Autodesk Fusion 360 part; units mm, degrees
(part 7 of 10)
sketch "草图24 (3)" plane through (0, 0, 0) normal (0, 0, 1) x (1, 0, 0) in component "R2_Integrated"
  line L0 (729, 50) -> (737, 50)
  line L1 (737, 50) -> (737, 131)
  line L2 (737, 131) -> (729, 131)
  line L3 (729, 131) -> (729, 50)
  dimension "d2854" = 729
  dimension "d2855" = 50
  dimension "d2856" = 8
  dimension "d2857" = 81
  constraint horizontal L0
  constraint vertical L1
  constraint horizontal L2
  constraint vertical L3
  measures "d2854" horizontal distance of origin L0.start
  measures "d2855" vertical distance of origin L0.start
  measures "d2856" horizontal distance of L0.start L0.end
  measures "d2857" vertical distance of L0.end L1.end
extrude "R03 integral runner 0''" add sketch "草图24 (3)" along normal blind 20 bodies 19 in component "R2_Integrated"
ref_plane "工作平面25" through (0, 0, 0) normal (0, 0, 1) x (1, 0, 0) in component "R2_Integrated"
sketch "草图25 (3)" plane through (0, 0, 0) normal (0, 0, 1) x (1, 0, 0) in component "R2_Integrated"
  line L0 (849, 50) -> (857, 50)
  line L1 (857, 50) -> (857, 131)
  line L2 (857, 131) -> (849, 131)
  line L3 (849, 131) -> (849, 50)
  dimension "d2862" = 849
  dimension "d2863" = 50
  dimension "d2864" = 8
  dimension "d2865" = 81
  constraint horizontal L0
  constraint vertical L1
  constraint horizontal L2
  constraint vertical L3
  measures "d2862" horizontal distance of origin L0.start
  measures "d2863" vertical distance of origin L0.start
  measures "d2864" horizontal distance of L0.start L0.end
  measures "d2865" vertical distance of L0.end L1.end
extrude "R03 integral runner 1''" add sketch "草图25 (3)" along normal blind 20 bodies 19 in component "R2_Integrated"
chamfer "R03 touch edge chamfer'''" distance 0.4 angle 45 5 edges at (729, 102.5, 40) (793, 53, 40) (857, 102.5, 40) (726, 95, 40) (860, 95, 40) on bodies 19 in component "R2_Integrated"
ref_plane "工作平面20" through (0, 0, 20) normal (0, 0, 1) x (1, 0, 0) in component "LS_Integrated"
sketch "草图20 (7)" plane through (0, 0, 20) normal (0, 0, 1) x (1, 0, 0) in component "LS_Integrated"
  line L0 (56.75, 306.75) -> (65.25, 306.75)
  line L1 (65.25, 306.75) -> (65.25, 315.25)
  line L2 (65.25, 315.25) -> (56.75, 315.25)
  line L3 (56.75, 315.25) -> (56.75, 306.75)
  dimension "d2871" = 56.75
  dimension "d2872" = 306.75
  dimension "d2873" = 8.5
  dimension "d2874" = 8.5
  constraint horizontal L0
  constraint vertical L1
  constraint horizontal L2
  constraint vertical L3
  measures "d2871" horizontal distance of origin L0.start
  measures "d2872" vertical distance of origin L0.start
  measures "d2873" horizontal distance of L0.start L0.end
  measures "d2874" vertical distance of L0.end L1.end
extrude "R03 fill obsolete socket 00''''" add sketch "草图20 (7)" along normal blind 1.8 bodies 25 in component "LS_Integrated"
ref_plane "工作平面21" through (0, 0, 20) normal (0, 0, 1) x (1, 0, 0) in component "LS_Integrated"
sketch "草图21 (7)" plane through (0, 0, 20) normal (0, 0, 1) x (1, 0, 0) in component "LS_Integrated"
  line L0 (148.75, 306.75) -> (157.25, 306.75)
  line L1 (157.25, 306.75) -> (157.25, 315.25)
  line L2 (157.25, 315.25) -> (148.75, 315.25)
  line L3 (148.75, 315.25) -> (148.75, 306.75)
  dimension "d2879" = 148.75
  dimension "d2880" = 306.75
  dimension "d2881" = 8.5
  dimension "d2882" = 8.5
  constraint horizontal L0
  constraint vertical L1
  constraint horizontal L2
  constraint vertical L3
  measures "d2879" horizontal distance of origin L0.start
  measures "d2880" vertical distance of origin L0.start
  measures "d2881" horizontal distance of L0.start L0.end
  measures "d2882" vertical distance of L0.end L1.end
extrude "R03 fill obsolete socket 01''''" add sketch "草图21 (7)" along normal blind 1.8 bodies 25 in component "LS_Integrated"
ref_plane "工作平面22" through (0, 0, 20) normal (0, 0, 1) x (1, 0, 0) in component "LS_Integrated"
sketch "草图22 (6)" plane through (0, 0, 20) normal (0, 0, 1) x (1, 0, 0) in component "LS_Integrated"
  line L0 (56.75, 148.75) -> (65.25, 148.75)
  line L1 (65.25, 148.75) -> (65.25, 157.25)
  line L2 (65.25, 157.25) -> (56.75, 157.25)
  line L3 (56.75, 157.25) -> (56.75, 148.75)
  dimension "d2887" = 56.75
  dimension "d2888" = 148.75
  dimension "d2889" = 8.5
  dimension "d2890" = 8.5
  constraint horizontal L0
  constraint vertical L1
  constraint horizontal L2
  constraint vertical L3
  measures "d2887" horizontal distance of origin L0.start
  measures "d2888" vertical distance of origin L0.start
  measures "d2889" horizontal distance of L0.start L0.end
  measures "d2890" vertical distance of L0.end L1.end
extrude "R03 fill obsolete socket 10''''" add sketch "草图22 (6)" along normal blind 1.8 bodies 25 in component "LS_Integrated"
ref_plane "工作平面23" through (0, 0, 20) normal (0, 0, 1) x (1, 0, 0) in component "LS_Integrated"
sketch "草图23 (6)" plane through (0, 0, 20) normal (0, 0, 1) x (1, 0, 0) in component "LS_Integrated"
  line L0 (148.75, 148.75) -> (157.25, 148.75)
  line L1 (157.25, 148.75) -> (157.25, 157.25)
  line L2 (157.25, 157.25) -> (148.75, 157.25)
  line L3 (148.75, 157.25) -> (148.75, 148.75)
  dimension "d2895" = 148.75
  dimension "d2896" = 148.75
  dimension "d2897" = 8.5
  dimension "d2898" = 8.5
  constraint horizontal L0
  constraint vertical L1
  constraint horizontal L2
  constraint vertical L3
  measures "d2895" horizontal distance of origin L0.start
  measures "d2896" vertical distance of origin L0.start
  measures "d2897" horizontal distance of L0.start L0.end
  measures "d2898" vertical distance of L0.end L1.end
extrude "R03 fill obsolete socket 11''''" add sketch "草图23 (6)" along normal blind 1.8 bodies 25 in component "LS_Integrated"
ref_plane "工作平面24" through (0, 0, 0) normal (0, 0, 1) x (1, 0, 0) in component "LS_Integrated"
sketch "草图24 (4)" plane through (0, 0, 0) normal (0, 0, 1) x (1, 0, 0) in component "LS_Integrated"
  line L0 (50, 311) -> (161, 311)
  line L1 (161, 311) -> (161, 319)
  line L2 (161, 319) -> (50, 319)
  line L3 (50, 319) -> (50, 311)
  dimension "d2903" = 50
  dimension "d2904" = 311
  dimension "d2905" = 111
  dimension "d2906" = 8
  constraint horizontal L0
  constraint vertical L1
  constraint horizontal L2
  constraint vertical L3
  measures "d2903" horizontal distance of origin L0.start
  measures "d2904" vertical distance of origin L0.start
  measures "d2905" horizontal distance of L0.start L0.end
  measures "d2906" vertical distance of L0.end L1.end
extrude "R03 integral runner 0'''" add sketch "草图24 (4)" along normal blind 20 bodies 25 in component "LS_Integrated"
ref_plane "工作平面25" through (0, 0, 0) normal (0, 0, 1) x (1, 0, 0) in component "LS_Integrated"
sketch "草图25 (4)" plane through (0, 0, 0) normal (0, 0, 1) x (1, 0, 0) in component "LS_Integrated"
  line L0 (50, 145) -> (161, 145)
  line L1 (161, 145) -> (161, 153)
  line L2 (161, 153) -> (50, 153)
  line L3 (50, 153) -> (50, 145)
  dimension "d2911" = 50
  dimension "d2912" = 145
  dimension "d2913" = 111
  dimension "d2914" = 8
  constraint horizontal L0
  constraint vertical L1
  constraint horizontal L2
  constraint vertical L3
  measures "d2911" horizontal distance of origin L0.start
  measures "d2912" vertical distance of origin L0.start
  measures "d2913" horizontal distance of L0.start L0.end
  measures "d2914" vertical distance of L0.end L1.end
extrude "R03 integral runner 1'''" add sketch "草图25 (4)" along normal blind 20 bodies 25 in component "LS_Integrated"
chamfer "R03 touch edge chamfer''''" distance 0.4 angle 45 5 edges at (117.5, 145, 40) (117.5, 319, 40) (110, 322, 40) (110, 142, 40) (53, 232, 40) on bodies 25 in component "LS_Integrated"
ref_plane "工作平面20" through (0, 0, 20) normal (0, 0, 1) x (1, 0, 0) in component "RS_Integrated"
sketch "草图20 (8)" plane through (0, 0, 20) normal (0, 0, 1) x (1, 0, 0) in component "RS_Integrated"
  line L0 (844.75, 148.75) -> (853.25, 148.75)
  line L1 (853.25, 148.75) -> (853.25, 157.25)
  line L2 (853.25, 157.25) -> (844.75, 157.25)
  line L3 (844.75, 157.25) -> (844.75, 148.75)
  dimension "d2920" = 844.75
  dimension "d2921" = 148.75
  dimension "d2922" = 8.5
  dimension "d2923" = 8.5
  constraint horizontal L0
  constraint vertical L1
  constraint horizontal L2
  constraint vertical L3
  measures "d2920" horizontal distance of origin L0.start
  measures "d2921" vertical distance of origin L0.start
  measures "d2922" horizontal distance of L0.start L0.end
  measures "d2923" vertical distance of L0.end L1.end
extrude "R03 fill obsolete socket 00'''''" add sketch "草图20 (8)" along normal blind 1.8 bodies 31 in component "RS_Integrated"
ref_plane "工作平面21" through (0, 0, 20) normal (0, 0, 1) x (1, 0, 0) in component "RS_Integrated"
sketch "草图21 (8)" plane through (0, 0, 20) normal (0, 0, 1) x (1, 0, 0) in component "RS_Integrated"
  line L0 (782.75, 148.75) -> (791.25, 148.75)
  line L1 (791.25, 148.75) -> (791.25, 157.25)
  line L2 (791.25, 157.25) -> (782.75, 157.25)
  line L3 (782.75, 157.25) -> (782.75, 148.75)
  dimension "d2928" = 782.75
  dimension "d2929" = 148.75
  dimension "d2930" = 8.5
  dimension "d2931" = 8.5
  constraint horizontal L0
  constraint vertical L1
  constraint horizontal L2
  constraint vertical L3
  measures "d2928" horizontal distance of origin L0.start
  measures "d2929" vertical distance of origin L0.start
  measures "d2930" horizontal distance of L0.start L0.end
  measures "d2931" vertical distance of L0.end L1.end
extrude "R03 fill obsolete socket 01'''''" add sketch "草图21 (8)" along normal blind 1.8 bodies 31 in component "RS_Integrated"
ref_plane "工作平面22" through (0, 0, 20) normal (0, 0, 1) x (1, 0, 0) in component "RS_Integrated"
sketch "草图22 (7)" plane through (0, 0, 20) normal (0, 0, 1) x (1, 0, 0) in component "RS_Integrated"
  line L0 (844.75, 306.75) -> (853.25, 306.75)
  line L1 (853.25, 306.75) -> (853.25, 315.25)
  line L2 (853.25, 315.25) -> (844.75, 315.25)
  line L3 (844.75, 315.25) -> (844.75, 306.75)
  dimension "d2936" = 844.75
  dimension "d2937" = 306.75
  dimension "d2938" = 8.5
  dimension "d2939" = 8.5
  constraint horizontal L0
  constraint vertical L1
  constraint horizontal L2
  constraint vertical L3
  measures "d2936" horizontal distance of origin L0.start
  measures "d2937" vertical distance of origin L0.start
  measures "d2938" horizontal distance of L0.start L0.end
  measures "d2939" vertical distance of L0.end L1.end
extrude "R03 fill obsolete socket 10'''''" add sketch "草图22 (7)" along normal blind 1.8 bodies 31 in component "RS_Integrated"
ref_plane "工作平面23" through (0, 0, 20) normal (0, 0, 1) x (1, 0, 0) in component "RS_Integrated"
sketch "草图23 (7)" plane through (0, 0, 20) normal (0, 0, 1) x (1, 0, 0) in component "RS_Integrated"
  line L0 (782.75, 306.75) -> (791.25, 306.75)
  line L1 (791.25, 306.75) -> (791.25, 315.25)
  line L2 (791.25, 315.25) -> (782.75, 315.25)
  line L3 (782.75, 315.25) -> (782.75, 306.75)
  dimension "d2944" = 782.75
  dimension "d2945" = 306.75
  dimension "d2946" = 8.5
  dimension "d2947" = 8.5
  constraint horizontal L0
  constraint vertical L1
  constraint horizontal L2
  constraint vertical L3
  measures "d2944" horizontal distance of origin L0.start
  measures "d2945" vertical distance of origin L0.start
  measures "d2946" horizontal distance of L0.start L0.end
  measures "d2947" vertical distance of L0.end L1.end
extrude "R03 fill obsolete socket 11'''''" add sketch "草图23 (7)" along normal blind 1.8 bodies 31 in component "RS_Integrated"
ref_plane "工作平面24" through (0, 0, 0) normal (0, 0, 1) x (1, 0, 0) in component "RS_Integrated"
sketch "草图24 (5)" plane through (0, 0, 0) normal (0, 0, 1) x (1, 0, 0) in component "RS_Integrated"
  line L0 (779, 145) -> (860, 145)
  line L1 (860, 145) -> (860, 153)
  line L2 (860, 153) -> (779, 153)
  line L3 (779, 153) -> (779, 145)
  dimension "d2952" = 779
  dimension "d2953" = 145
  dimension "d2954" = 81
  dimension "d2955" = 8
  constraint horizontal L0
  constraint vertical L1
  constraint horizontal L2
  constraint vertical L3
  measures "d2952" horizontal distance of origin L0.start
  measures "d2953" vertical distance of origin L0.start
  measures "d2954" horizontal distance of L0.start L0.end
  measures "d2955" vertical distance of L0.end L1.end
extrude "R03 integral runner 0''''" add sketch "草图24 (5)" along normal blind 20 bodies 31 in component "RS_Integrated"
ref_plane "工作平面25" through (0, 0, 0) normal (0, 0, 1) x (1, 0, 0) in component "RS_Integrated"
sketch "草图25 (5)" plane through (0, 0, 0) normal (0, 0, 1) x (1, 0, 0) in component "RS_Integrated"
  line L0 (779, 311) -> (860, 311)
  line L1 (860, 311) -> (860, 319)
  line L2 (860, 319) -> (779, 319)
  line L3 (779, 319) -> (779, 311)
  dimension "d2960" = 779
  dimension "d2961" = 311
  dimension "d2962" = 81
  dimension "d2963" = 8
  constraint horizontal L0
  constraint vertical L1
  constraint horizontal L2
  constraint vertical L3
  measures "d2960" horizontal distance of origin L0.start
  measures "d2961" vertical distance of origin L0.start
  measures "d2962" horizontal distance of L0.start L0.end
  measures "d2963" vertical distance of L0.end L1.end
extrude "R03 integral runner 1''''" add sketch "草图25 (5)" along normal blind 20 bodies 31 in component "RS_Integrated"
chamfer "R03 touch edge chamfer'''''" distance 0.4 angle 45 5 edges at (807.5, 319, 40) (807.5, 145, 40) (857, 232, 40) (815, 142, 40) (815, 322, 40) on bodies 31 in component "RS_Integrated"
chamfer "R03 touch edge chamfer''''''" distance 0.4 angle 45 5 edges at (63.3, 101, 40) (216.7, 101, 40) (182.35, 136.7, 40) (97.65, 136.7, 40) (140, 53.3, 40) on bodies 2 in component "L1_RemovableGrate"
chamfer "R03 touch edge chamfer'''''''" distance 0.4 angle 45 5 edges at (235.3, 101, 40) (426.7, 101, 40) (382.85, 136.7, 40) (279.15, 136.7, 40) (331, 53.3, 40) on bodies 8 in component "L2_RemovableGrate"
chamfer "R03 touch edge chamfer''''''''" distance 0.4 angle 45 5 edges at (593.3, 101, 40) (720.7, 101, 40) (692.85, 136.7, 40) (621.15, 136.7, 40) (657, 53.3, 40) on bodies 14 in component "R1_RemovableGrate"
chamfer "R03 touch edge chamfer'''''''''" distance 0.4 angle 45 5 edges at (729.3, 101, 40) (856.7, 101, 40) (828.85, 136.7, 40) (757.15, 136.7, 40) (793, 53.3, 40) on bodies 20 in component "R2_RemovableGrate"
chamfer "R03 touch edge chamfer''''''''''" distance 0.4 angle 45 5 edges at (116, 318.7, 40) (166.7, 184.65, 40) (166.7, 279.35, 40) (116, 145.3, 40) (53.3, 232, 40) on bodies 26 in component "LS_RemovableGrate"
chamfer "R03 touch edge chamfer'''''''''''" distance 0.4 angle 45 5 edges at (809, 318.7, 40) (773.3, 279.35, 40) (773.3, 184.65, 40) (809, 145.3, 40) (856.7, 232, 40) on bodies 32 in component "RS_RemovableGrate"
chamfer "R03 touch edge chamfer''''''''''''" distance 0.4 angle 45 5 edges at (53.3, 102.5, 145) (226.7, 102.5, 145) (187.35, 136.7, 145) (92.65, 136.7, 145) (140, 53.3, 145) on bodies 38 in component "UP_RemovableGrate"
component "L1_DrainPan" placed x (1, 0, 0) y (0, 1, 0) z (0, 0, 1) at (0, 0, 0)
component "L1_RemovableGrate" placed x (1, 0, 0) y (0, 1, 0) z (0, 0, 1) at (0, 0, 0)
component "L2_Integrated" placed x (1, 0, 0) y (0, 1, 0) z (0, 0, 1) at (0, 0, 0)
component "L2_RemovableGrate" placed x (1, 0, 0) y (0, 1, 0) z (0, 0, 1) at (0, 0, 0)
component "R1_Integrated" placed x (1, 0, 0) y (0, 1, 0) z (0, 0, 1) at (0, 0, 0)
component "R1_RemovableGrate" placed x (1, 0, 0) y (0, 1, 0) z (0, 0, 1) at (0, 0, 0)
component "R2_Integrated" placed x (1, 0, 0) y (0, 1, 0) z (0, 0, 1) at (0, 0, 0)
component "R2_RemovableGrate" placed x (1, 0, 0) y (0, 1, 0) z (0, 0, 1) at (0, 0, 0)
component "LS_Integrated" placed x (1, 0, 0) y (0, 1, 0) z (0, 0, 1) at (0, 0, 0)
component "LS_RemovableGrate" placed x (1, 0, 0) y (0, 1, 0) z (0, 0, 1) at (0, 0, 0)
component "RS_Integrated" placed x (1, 0, 0) y (0, 1, 0) z (0, 0, 1) at (0, 0, 0)
component "RS_RemovableGrate" placed x (1, 0, 0) y (0, 1, 0) z (0, 0, 1) at (0, 0, 0)
component "Tower_Integrated" placed x (1, 0, 0) y (0, 1, 0) z (0, 0, 1) at (0, 0, 0)
component "UP_RemovableGrate" placed x (1, 0, 0) y (0, 1, 0) z (0, 0, 1) at (0, 0, 0)
equation "LeftAvailable = 400 mm" comment "User approximate dimension: left of faucet"
equation "RightAvailable = 300 mm" comment "User approximate dimension: right of faucet"
equation "RearAvailable = 100 mm" comment "User approximate rear strip depth"
equation "LeftSideAvailable = 130 mm" comment "User approximate left strip width"
equation "MirrorClearance = 300 mm" comment "User approximate countertop to mirror cabinet"
equation "RightSideAvailable = 100 mm" comment "ASSUMPTION: awaiting measurement"
equation "LeftReach = 180 mm" comment "ASSUMPTION: forward side extension beyond rear rack"
equation "RightReach = 180 mm" comment "ASSUMPTION: forward side extension beyond rear rack"
equation "FaucetGap = 160 mm" comment "ASSUMPTION: faucet and lever clearance, awaiting measurement"
equation "LeftRun = LeftAvailable - 20 mm" comment "Design clearance allowance; check on site"
equation "RightRun = RightAvailable - 30 mm" comment "Design clearance allowance; check lever"
equation "Depth = RearAvailable - 10 mm" comment "Rear standing module depth"
equation "LeftSideDepth = LeftSideAvailable - 10 mm" comment "Left side module depth"
equation "RightSideDepth = RightSideAvailable - 10 mm" comment "Right side module depth, provisional"
equation "ModuleGap = 2 mm" comment "Open cleaning / assembly seam, not watertight"
equation "TowerWidth = 180 mm" comment "Local upper tier only"
equation "TowerFrame = 8 mm" comment "Side portal frame thickness"
equation "TowerClearance = 2 mm" comment "Clearance from lower tray to side frames"
equation "FootHeight = 20 mm" comment "Clear gap below pan"
equation "PanHeight = 20 mm" comment "Pan rim above underside"
equation "FloorMin = 3 mm" comment "Minimum pan floor at outlet"
equation "Wall = 3 mm" comment "Pan walls"
equation "DrainSlope = 4 deg" comment "Initial design slope; verify with water test"
equation "DeckThick = 4 mm" comment "Removable horizontal grate thickness"
equation "DeckClearance = 0.3 mm" comment "Per-side clearance; fit coupon required"
equation "RimBorder = 7 mm" comment "Solid grate border"
equation "SlotWidth = 4 mm" comment "Open slat gaps"
equation "SlotPitch = 10 mm" comment "Initial grate slot spacing"
equation "DrainWidth = 28 mm" comment "R01 construction history only: R02 opens the entire front between side walls"
equation "DrainExtension = 25 mm" comment "R01 construction parameter: R02 has no external projection; this value still contributes to inherited floor thickness"
equation "UpperDeckHeight = 145 mm" comment "Small jars only; verify cabinet swing"
equation "FootSize = 16 mm" comment "Support foot footprint"
equation "PegSize = 8 mm" comment "Square locating peg"
equation "PegHeight = 1.5 mm" comment "Foot locating peg, not a locking fastener"
equation "FitClearance = 0.25 mm" comment "Per-side foot fit allowance; test first"
equation "BaseX = 50 mm" comment "Model datum offset"
equation "BaseY = 50 mm" comment "Model datum offset"
equation "d38 = FootHeight"
equation "d40 = ( BaseX + TowerFrame + TowerClearance ) + ( 0 mm )"
equation "d41 = ( BaseY ) + ( 0 mm )"
equation "d42 = TowerWidth - 2 * ( TowerFrame + TowerClearance )"
equation "d43 = Depth"
equation "d44 = PanHeight"
equation "d48 = ( BaseX + TowerFrame + TowerClearance ) + ( Wall )"
equation "d50 = -( -( ( FootHeight ) + FloorMin + DrainExtension * tan(DrainSlope) + ( ( Depth ) - ( Wall ) ) * tan(DrainSlope) ) )"
equation "d51 = ( ( BaseY ) + ( Wall ) )"
equation "d52 = -( -( ( FootHeight ) + FloorMin + DrainExtension * tan(DrainSlope) + ( ( Depth ) - ( ( Depth ) - Wall ) ) * tan(DrainSlope) ) )"
equation "d53 = ( ( BaseY ) + ( ( Depth ) - Wall ) )"
equation "d54 = -( -( ( FootHeight ) + PanHeight + 1 mm ) )"
equation "d55 = ( TowerWidth - 2 * ( TowerFrame + TowerClearance ) ) - 2 * Wall"
equation "d57 = ( BaseX + TowerFrame + TowerClearance ) + ( ( TowerWidth - 2 * ( TowerFrame + TowerClearance ) - 31 mm ) - DrainWidth / 2 - Wall )"
equation "d59 = -( -( FootHeight ) )"
equation "d60 = ( ( BaseY ) + ( ( Depth ) - Wall ) )"
equation "d61 = ( ( BaseY ) + ( ( Depth ) + DrainExtension ) )"
equation "d62 = -( -( ( FootHeight ) + FloorMin + DrainExtension * tan(DrainSlope) + ( ( Depth ) - ( ( Depth ) + DrainExtension ) ) * tan(DrainSlope) ) )"
equation "d63 = -( -( ( FootHeight ) + FloorMin + DrainExtension * tan(DrainSlope) + ( ( Depth ) - ( ( Depth ) - Wall ) ) * tan(DrainSlope) ) )"
equation "d64 = DrainWidth + 2 * Wall"
equation "d66 = ( BaseX + TowerFrame + TowerClearance ) + ( ( TowerWidth - 2 * ( TowerFrame + TowerClearance ) - 31 mm ) - DrainWidth / 2 - Wall )"
equation "d68 = -( -( FootHeight ) )"
equation "d69 = ( ( BaseY ) + ( ( Depth ) - Wall ) )"
equation "d70 = ( ( BaseY ) + ( ( Depth ) + DrainExtension ) )"
equation "d71 = -( -( ( ( FootHeight ) + FloorMin + DrainExtension * tan(DrainSlope) + ( ( Depth ) - ( ( Depth ) + DrainExtension ) ) * tan(DrainSlope) ) + ( 6 mm ) ) )"
equation "d72 = -( -( ( ( FootHeight ) + FloorMin + DrainExtension * tan(DrainSlope) + ( ( Depth ) - ( ( Depth ) - Wall ) ) * tan(DrainSlope) ) + ( 6 mm ) ) )"
equation "d73 = Wall"
equation "d75 = ( BaseX + TowerFrame + TowerClearance ) + ( ( TowerWidth - 2 * ( TowerFrame + TowerClearance ) - 31 mm ) + DrainWidth / 2 )"
equation "d77 = -( -( FootHeight ) )"
equation "d78 = ( ( BaseY ) + ( ( Depth ) - Wall ) )"
equation "d79 = ( ( BaseY ) + ( ( Depth ) + DrainExtension ) )"
equation "d80 = -( -( ( ( FootHeight ) + FloorMin + DrainExtension * tan(DrainSlope) + ( ( Depth ) - ( ( Depth ) + DrainExtension ) ) * tan(DrainSlope) ) + ( 6 mm ) ) )"
equation "d81 = -( -( ( ( FootHeight ) + FloorMin + DrainExtension * tan(DrainSlope) + ( ( Depth ) - ( ( Depth ) - Wall ) ) * tan(DrainSlope) ) + ( 6 mm ) ) )"
equation "d82 = Wall"
equation "d84 = ( BaseX + TowerFrame + TowerClearance ) + ( ( TowerWidth - 2 * ( TowerFrame + TowerClearance ) - 31 mm ) - DrainWidth / 2 )"
equation "d86 = -( -( ( FootHeight ) + FloorMin + DrainExtension * tan(DrainSlope) + ( ( Depth ) - ( ( Depth ) - Wall ) ) * tan(DrainSlope) ) )"
equation "d87 = ( ( BaseY ) + ( ( Depth ) - Wall ) )"
equation "d88 = -( -( ( FootHeight ) + FloorMin + DrainExtension * tan(DrainSlope) + ( ( Depth ) - ( ( Depth ) + DrainExtension ) ) * tan(DrainSlope) ) )"
equation "d89 = ( ( BaseY ) + ( ( Depth ) + DrainExtension ) )"
equation "d90 = -( -( ( FootHeight ) + PanHeight + 1 mm ) )"
equation "d91 = DrainWidth"
equation "d93 = FootHeight"
equation "d95 = ( BaseX + TowerFrame + TowerClearance ) + ( Wall )"
equation "d96 = ( BaseY ) + ( Wall )"
equation "d99 = PanHeight - DeckThick"
equation "d101 = FootHeight"
equation "d103 = ( BaseX + TowerFrame + TowerClearance ) + ( Wall )"
equation "d104 = ( BaseY ) + ( ( Depth ) - Wall - 12 mm )"
equation "d107 = PanHeight - DeckThick"
equation "d109 = FootHeight"
equation "d111 = ( BaseX + TowerFrame + TowerClearance ) + ( ( TowerWidth - 2 * ( TowerFrame + TowerClearance ) ) - Wall - 12 mm )"
equation "d112 = ( BaseY ) + ( Wall )"
equation "d115 = PanHeight - DeckThick"
equation "d117 = FootHeight"
equation "d119 = ( BaseX + TowerFrame + TowerClearance ) + ( ( TowerWidth - 2 * ( TowerFrame + TowerClearance ) ) - Wall - 12 mm )"
equation "d120 = ( BaseY ) + ( ( Depth ) - Wall - 12 mm )"
equation "d123 = PanHeight - DeckThick"
equation "d125 = ( BaseX + TowerFrame + TowerClearance ) + ( ( TowerWidth - 2 * ( TowerFrame + TowerClearance ) - 31 mm ) - DrainWidth / 2 - Wall )"
equation "d127 = -( -( ( FootHeight ) - ( 0.2 mm ) ) )"
equation "d128 = ( ( BaseY ) + ( ( Depth ) + DrainExtension - 2 mm ) )"
equation "d129 = ( ( BaseY ) + ( ( ( Depth ) + DrainExtension - 2 mm ) + ( 1 mm ) ) )"
equation "d130 = -( -( ( FootHeight ) + ( 0.6 mm ) ) )"
equation "d131 = DrainWidth + 2 * Wall"
equation "d133 = FootHeight"
equation "d135 = ( BaseX + TowerFrame + TowerClearance ) + ( ( 11 mm ) - PegSize / 2 - FitClearance )"
equation "d136 = ( BaseY ) + ( ( 11 mm ) - PegSize / 2 - FitClearance )"
equation "d137 = PegSize + 2 * FitClearance"
equation "d138 = PegSize + 2 * FitClearance"
equation "d139 = PegHeight + 0.3 mm"
equation "d141 = FootHeight"
equation "d143 = ( BaseX + TowerFrame + TowerClearance ) + ( ( 11 mm ) - PegSize / 2 - FitClearance )"
equation "d144 = ( BaseY ) + ( ( ( Depth ) - FrontFootInset ) - PegSize / 2 - FitClearance )"
equation "d145 = PegSize + 2 * FitClearance"
equation "d146 = PegSize + 2 * FitClearance"
equation "d147 = PegHeight + 0.3 mm"
equation "d149 = FootHeight"
equation "d151 = ( BaseX + TowerFrame + TowerClearance ) + ( ( ( TowerWidth - 2 * ( TowerFrame + TowerClearance ) ) - 11 mm ) - PegSize / 2 - FitClearance )"
equation "d152 = ( BaseY ) + ( ( 11 mm ) - PegSize / 2 - FitClearance )"
equation "d153 = PegSize + 2 * FitClearance"
equation "d154 = PegSize + 2 * FitClearance"
equation "d155 = PegHeight + 0.3 mm"
equation "d157 = FootHeight"
equation "d159 = ( BaseX + TowerFrame + TowerClearance ) + ( ( ( TowerWidth - 2 * ( TowerFrame + TowerClearance ) ) - 11 mm ) - PegSize / 2 - FitClearance )"
equation "d160 = ( BaseY ) + ( ( ( Depth ) - FrontFootInset ) - PegSize / 2 - FitClearance )"
equation "d161 = PegSize + 2 * FitClearance"
equation "d162 = PegSize + 2 * FitClearance"
equation "d163 = PegHeight + 0.3 mm"
equation "d165 = ( FootHeight ) + PanHeight - DeckThick"
equation "d167 = ( BaseX + TowerFrame + TowerClearance ) + ( Wall + DeckClearance )"
equation "d168 = ( BaseY ) + ( Wall + DeckClearance )"
equation "d169 = ( TowerWidth - 2 * ( TowerFrame + TowerClearance ) ) - 2 * ( Wall + DeckClearance )"
equation "d170 = ( Depth ) - 2 * ( Wall + DeckClearance )"
equation "d171 = DeckThick"
equation "d173 = ( FootHeight ) + PanHeight - DeckThick"
equation "d175 = ( BaseX + TowerFrame + TowerClearance ) + ( ( ( ( TowerWidth - 2 * ( TowerFrame + TowerClearance ) ) - ( 12 * SlotPitch + SlotWidth ) ) / 2 ) + ( 0 * SlotPitch ) )"
equation "d176 = ( BaseY ) + ( Wall + DeckClearance + RimBorder )"
equation "d177 = SlotWidth"
equation "d178 = ( Depth ) - 2 * ( Wall + DeckClearance + RimBorder )"
equation "d179 = DeckThick"
equation "d181 = ( FootHeight ) + PanHeight - DeckThick"
equation "d183 = ( BaseX + TowerFrame + TowerClearance ) + ( ( ( ( TowerWidth - 2 * ( TowerFrame + TowerClearance ) ) - ( 12 * SlotPitch + SlotWidth ) ) / 2 ) + ( 1 * SlotPitch ) )"
equation "d184 = ( BaseY ) + ( Wall + DeckClearance + RimBorder )"
equation "d185 = SlotWidth"
equation "d186 = ( Depth ) - 2 * ( Wall + DeckClearance + RimBorder )"
equation "d187 = DeckThick"
equation "d189 = ( FootHeight ) + PanHeight - DeckThick"
equation "d191 = ( BaseX + TowerFrame + TowerClearance ) + ( ( ( ( TowerWidth - 2 * ( TowerFrame + TowerClearance ) ) - ( 12 * SlotPitch + SlotWidth ) ) / 2 ) + ( 2 * SlotPitch ) )"
equation "d192 = ( BaseY ) + ( Wall + DeckClearance + RimBorder )"
equation "d193 = SlotWidth"
equation "d194 = ( Depth ) - 2 * ( Wall + DeckClearance + RimBorder )"
equation "d195 = DeckThick"
equation "d197 = ( FootHeight ) + PanHeight - DeckThick"
equation "d199 = ( BaseX + TowerFrame + TowerClearance ) + ( ( ( ( TowerWidth - 2 * ( TowerFrame + TowerClearance ) ) - ( 12 * SlotPitch + SlotWidth ) ) / 2 ) + ( 3 * SlotPitch ) )"
equation "d200 = ( BaseY ) + ( Wall + DeckClearance + RimBorder )"
equation "d201 = SlotWidth"
equation "d202 = ( Depth ) - 2 * ( Wall + DeckClearance + RimBorder )"
equation "d203 = DeckThick"
equation "d205 = ( FootHeight ) + PanHeight - DeckThick"
equation "d207 = ( BaseX + TowerFrame + TowerClearance ) + ( ( ( ( TowerWidth - 2 * ( TowerFrame + TowerClearance ) ) - ( 12 * SlotPitch + SlotWidth ) ) / 2 ) + ( 4 * SlotPitch ) )"
equation "d208 = ( BaseY ) + ( Wall + DeckClearance + RimBorder )"
equation "d209 = SlotWidth"
equation "d210 = ( Depth ) - 2 * ( Wall + DeckClearance + RimBorder )"
equation "d211 = DeckThick"
equation "d213 = ( FootHeight ) + PanHeight - DeckThick"
equation "d215 = ( BaseX + TowerFrame + TowerClearance ) + ( ( ( ( TowerWidth - 2 * ( TowerFrame + TowerClearance ) ) - ( 12 * SlotPitch + SlotWidth ) ) / 2 ) + ( 5 * SlotPitch ) )"
equation "d216 = ( BaseY ) + ( Wall + DeckClearance + RimBorder )"
equation "d217 = SlotWidth"
equation "d218 = ( Depth ) - 2 * ( Wall + DeckClearance + RimBorder )"
equation "d219 = DeckThick"
equation "d221 = ( FootHeight ) + PanHeight - DeckThick"
equation "d223 = ( BaseX + TowerFrame + TowerClearance ) + ( ( ( ( TowerWidth - 2 * ( TowerFrame + TowerClearance ) ) - ( 12 * SlotPitch + SlotWidth ) ) / 2 ) + ( 6 * SlotPitch ) )"
equation "d224 = ( BaseY ) + ( Wall + DeckClearance + RimBorder )"
equation "d225 = SlotWidth"
equation "d226 = ( Depth ) - 2 * ( Wall + DeckClearance + RimBorder )"
equation "d227 = DeckThick"
equation "d229 = ( FootHeight ) + PanHeight - DeckThick"
equation "d231 = ( BaseX + TowerFrame + TowerClearance ) + ( ( ( ( TowerWidth - 2 * ( TowerFrame + TowerClearance ) ) - ( 12 * SlotPitch + SlotWidth ) ) / 2 ) + ( 7 * SlotPitch ) )"
equation "d232 = ( BaseY ) + ( Wall + DeckClearance + RimBorder )"
equation "d233 = SlotWidth"
equation "d234 = ( Depth ) - 2 * ( Wall + DeckClearance + RimBorder )"
equation "d235 = DeckThick"
equation "d237 = ( FootHeight ) + PanHeight - DeckThick"
equation "d239 = ( BaseX + TowerFrame + TowerClearance ) + ( ( ( ( TowerWidth - 2 * ( TowerFrame + TowerClearance ) ) - ( 12 * SlotPitch + SlotWidth ) ) / 2 ) + ( 8 * SlotPitch ) )"
equation "d240 = ( BaseY ) + ( Wall + DeckClearance + RimBorder )"
equation "d241 = SlotWidth"
equation "d242 = ( Depth ) - 2 * ( Wall + DeckClearance + RimBorder )"
equation "d243 = DeckThick"
equation "d245 = ( FootHeight ) + PanHeight - DeckThick"
equation "d247 = ( BaseX + TowerFrame + TowerClearance ) + ( ( ( ( TowerWidth - 2 * ( TowerFrame + TowerClearance ) ) - ( 12 * SlotPitch + SlotWidth ) ) / 2 ) + ( 9 * SlotPitch ) )"
equation "d248 = ( BaseY ) + ( Wall + DeckClearance + RimBorder )"
equation "d249 = SlotWidth"
equation "d250 = ( Depth ) - 2 * ( Wall + DeckClearance + RimBorder )"
equation "d251 = DeckThick"
equation "d253 = ( FootHeight ) + PanHeight - DeckThick"
equation "d255 = ( BaseX + TowerFrame + TowerClearance ) + ( ( ( ( TowerWidth - 2 * ( TowerFrame + TowerClearance ) ) - ( 12 * SlotPitch + SlotWidth ) ) / 2 ) + ( 10 * SlotPitch ) )"
equation "d256 = ( BaseY ) + ( Wall + DeckClearance + RimBorder )"
equation "d257 = SlotWidth"
equation "d258 = ( Depth ) - 2 * ( Wall + DeckClearance + RimBorder )"
equation "d259 = DeckThick"
equation "d261 = ( FootHeight ) + PanHeight - DeckThick"
equation "d263 = ( BaseX + TowerFrame + TowerClearance ) + ( ( ( ( TowerWidth - 2 * ( TowerFrame + TowerClearance ) ) - ( 12 * SlotPitch + SlotWidth ) ) / 2 ) + ( 11 * SlotPitch ) )"
equation "d264 = ( BaseY ) + ( Wall + DeckClearance + RimBorder )"
equation "d265 = SlotWidth"
equation "d266 = ( Depth ) - 2 * ( Wall + DeckClearance + RimBorder )"
equation "d267 = DeckThick"
equation "d269 = ( FootHeight ) + PanHeight - DeckThick"
equation "d271 = ( BaseX + TowerFrame + TowerClearance ) + ( ( ( ( TowerWidth - 2 * ( TowerFrame + TowerClearance ) ) - ( 12 * SlotPitch + SlotWidth ) ) / 2 ) + ( 12 * SlotPitch ) )"
equation "d272 = ( BaseY ) + ( Wall + DeckClearance + RimBorder )"
equation "d273 = SlotWidth"
equation "d274 = ( Depth ) - 2 * ( Wall + DeckClearance + RimBorder )"
equation "d275 = DeckThick"
equation "d277 = ( FootHeight ) + PanHeight - DeckThick"
equation "d279 = ( BaseX + TowerFrame + TowerClearance ) + ( ( TowerWidth - 2 * ( TowerFrame + TowerClearance ) ) / 2 - 8 mm )"
equation "d280 = ( BaseY ) + ( ( Depth ) - Wall - DeckClearance - 4 mm )"
equation "d283 = DeckThick"
equation "d287 = ( BaseX + TowerFrame + TowerClearance ) + ( ( 11 mm ) - FootSize / 2 )"
equation "d288 = ( BaseY ) + ( ( 11 mm ) - FootSize / 2 )"
equation "d289 = FootSize"
equation "d290 = FootSize"
equation "d291 = FootHeight"
equation "d293 = FootHeight"
equation "d295 = ( BaseX + TowerFrame + TowerClearance ) + ( ( 11 mm ) - PegSize / 2 )"
equation "d296 = ( BaseY ) + ( ( 11 mm ) - PegSize / 2 )"
equation "d297 = PegSize"
equation "d298 = PegSize"
equation "d299 = PegHeight"
equation "d303 = ( BaseX + TowerFrame + TowerClearance ) + ( ( 11 mm ) - FootSize / 2 )"
equation "d304 = ( BaseY ) + ( ( ( Depth ) - FrontFootInset ) - FootSize / 2 )"
equation "d305 = FootSize"
equation "d306 = FootSize"
equation "d307 = FootHeight"
equation "d309 = FootHeight"
equation "d311 = ( BaseX + TowerFrame + TowerClearance ) + ( ( 11 mm ) - PegSize / 2 )"
equation "d312 = ( BaseY ) + ( ( ( Depth ) - FrontFootInset ) - PegSize / 2 )"
equation "d313 = PegSize"
equation "d314 = PegSize"
equation "d315 = PegHeight"
equation "d319 = ( BaseX + TowerFrame + TowerClearance ) + ( ( ( TowerWidth - 2 * ( TowerFrame + TowerClearance ) ) - 11 mm ) - FootSize / 2 )"
equation "d320 = ( BaseY ) + ( ( 11 mm ) - FootSize / 2 )"
equation "d321 = FootSize"
equation "d322 = FootSize"
equation "d323 = FootHeight"
equation "d325 = FootHeight"
equation "d327 = ( BaseX + TowerFrame + TowerClearance ) + ( ( ( TowerWidth - 2 * ( TowerFrame + TowerClearance ) ) - 11 mm ) - PegSize / 2 )"
equation "d328 = ( BaseY ) + ( ( 11 mm ) - PegSize / 2 )"
equation "d329 = PegSize"
equation "d330 = PegSize"
equation "d331 = PegHeight"
equation "d335 = ( BaseX + TowerFrame + TowerClearance ) + ( ( ( TowerWidth - 2 * ( TowerFrame + TowerClearance ) ) - 11 mm ) - FootSize / 2 )"
equation "d336 = ( BaseY ) + ( ( ( Depth ) - FrontFootInset ) - FootSize / 2 )"
equation "d337 = FootSize"
equation "d338 = FootSize"
equation "d339 = FootHeight"
equation "d341 = FootHeight"
equation "d343 = ( BaseX + TowerFrame + TowerClearance ) + ( ( ( TowerWidth - 2 * ( TowerFrame + TowerClearance ) ) - 11 mm ) - PegSize / 2 )"
equation "d344 = ( BaseY ) + ( ( ( Depth ) - FrontFootInset ) - PegSize / 2 )"
equation "d345 = PegSize"
equation "d346 = PegSize"
equation "d347 = PegHeight"
equation "d349 = FootHeight"
equation "d351 = ( BaseX + TowerWidth + ModuleGap ) + ( 0 mm )"
equation "d352 = ( BaseY ) + ( 0 mm )"
equation "d353 = LeftRun - TowerWidth - ModuleGap"
equation "d354 = Depth"
equation "d355 = PanHeight"
equation "d359 = ( BaseX + TowerWidth + ModuleGap ) + ( Wall )"
equation "d361 = -( -( ( FootHeight ) + FloorMin + DrainExtension * tan(DrainSlope) + ( ( Depth ) - ( Wall ) ) * tan(DrainSlope) ) )"
equation "d362 = ( ( BaseY ) + ( Wall ) )"
equation "d363 = -( -( ( FootHeight ) + FloorMin + DrainExtension * tan(DrainSlope) + ( ( Depth ) - ( ( Depth ) - Wall ) ) * tan(DrainSlope) ) )"
equation "d364 = ( ( BaseY ) + ( ( Depth ) - Wall ) )"
equation "d365 = -( -( ( FootHeight ) + PanHeight + 1 mm ) )"
equation "d366 = ( LeftRun - TowerWidth - ModuleGap ) - 2 * Wall"
equation "d368 = ( BaseX + TowerWidth + ModuleGap ) + ( ( ( LeftRun - TowerWidth - ModuleGap ) / 2 ) - DrainWidth / 2 - Wall )"
equation "d370 = -( -( FootHeight ) )"
equation "d371 = ( ( BaseY ) + ( ( Depth ) - Wall ) )"
equation "d372 = ( ( BaseY ) + ( ( Depth ) + DrainExtension ) )"
equation "d373 = -( -( ( FootHeight ) + FloorMin + DrainExtension * tan(DrainSlope) + ( ( Depth ) - ( ( Depth ) + DrainExtension ) ) * tan(DrainSlope) ) )"
equation "d374 = -( -( ( FootHeight ) + FloorMin + DrainExtension * tan(DrainSlope) + ( ( Depth ) - ( ( Depth ) - Wall ) ) * tan(DrainSlope) ) )"
equation "d375 = DrainWidth + 2 * Wall"
equation "d377 = ( BaseX + TowerWidth + ModuleGap ) + ( ( ( LeftRun - TowerWidth - ModuleGap ) / 2 ) - DrainWidth / 2 - Wall )"
equation "d379 = -( -( FootHeight ) )"
equation "d380 = ( ( BaseY ) + ( ( Depth ) - Wall ) )"
equation "d381 = ( ( BaseY ) + ( ( Depth ) + DrainExtension ) )"
equation "d382 = -( -( ( ( FootHeight ) + FloorMin + DrainExtension * tan(DrainSlope) + ( ( Depth ) - ( ( Depth ) + DrainExtension ) ) * tan(DrainSlope) ) + ( 6 mm ) ) )"
equation "d383 = -( -( ( ( FootHeight ) + FloorMin + DrainExtension * tan(DrainSlope) + ( ( Depth ) - ( ( Depth ) - Wall ) ) * tan(DrainSlope) ) + ( 6 mm ) ) )"
equation "d384 = Wall"
equation "d386 = ( BaseX + TowerWidth + ModuleGap ) + ( ( ( LeftRun - TowerWidth - ModuleGap ) / 2 ) + DrainWidth / 2 )"
equation "d388 = -( -( FootHeight ) )"
equation "d389 = ( ( BaseY ) + ( ( Depth ) - Wall ) )"
equation "d390 = ( ( BaseY ) + ( ( Depth ) + DrainExtension ) )"
equation "d391 = -( -( ( ( FootHeight ) + FloorMin + DrainExtension * tan(DrainSlope) + ( ( Depth ) - ( ( Depth ) + DrainExtension ) ) * tan(DrainSlope) ) + ( 6 mm ) ) )"
equation "d392 = -( -( ( ( FootHeight ) + FloorMin + DrainExtension * tan(DrainSlope) + ( ( Depth ) - ( ( Depth ) - Wall ) ) * tan(DrainSlope) ) + ( 6 mm ) ) )"
equation "d393 = Wall"
equation "d395 = ( BaseX + TowerWidth + ModuleGap ) + ( ( ( LeftRun - TowerWidth - ModuleGap ) / 2 ) - DrainWidth / 2 )"
equation "d397 = -( -( ( FootHeight ) + FloorMin + DrainExtension * tan(DrainSlope) + ( ( Depth ) - ( ( Depth ) - Wall ) ) * tan(DrainSlope) ) )"
equation "d398 = ( ( BaseY ) + ( ( Depth ) - Wall ) )"
equation "d399 = -( -( ( FootHeight ) + FloorMin + DrainExtension * tan(DrainSlope) + ( ( Depth ) - ( ( Depth ) + DrainExtension ) ) * tan(DrainSlope) ) )"
equation "d400 = ( ( BaseY ) + ( ( Depth ) + DrainExtension ) )"
equation "d401 = -( -( ( FootHeight ) + PanHeight + 1 mm ) )"
equation "d402 = DrainWidth"
equation "d404 = FootHeight"
equation "d406 = ( BaseX + TowerWidth + ModuleGap ) + ( Wall )"
equation "d407 = ( BaseY ) + ( Wall )"
equation "d410 = PanHeight - DeckThick"
equation "d412 = FootHeight"
equation "d414 = ( BaseX + TowerWidth + ModuleGap ) + ( Wall )"
equation "d415 = ( BaseY ) + ( ( Depth ) - Wall - 12 mm )"
equation "d418 = PanHeight - DeckThick"
equation "d420 = FootHeight"
equation "d422 = ( BaseX + TowerWidth + ModuleGap ) + ( ( LeftRun - TowerWidth - ModuleGap ) - Wall - 12 mm )"
equation "d423 = ( BaseY ) + ( Wall )"
equation "d426 = PanHeight - DeckThick"
equation "d428 = FootHeight"
equation "d430 = ( BaseX + TowerWidth + ModuleGap ) + ( ( LeftRun - TowerWidth - ModuleGap ) - Wall - 12 mm )"
equation "d431 = ( BaseY ) + ( ( Depth ) - Wall - 12 mm )"
equation "d434 = PanHeight - DeckThick"
equation "d436 = ( BaseX + TowerWidth + ModuleGap ) + ( ( ( LeftRun - TowerWidth - ModuleGap ) / 2 ) - DrainWidth / 2 - Wall )"
equation "d438 = -( -( ( FootHeight ) - ( 0.2 mm ) ) )"
equation "d439 = ( ( BaseY ) + ( ( Depth ) + DrainExtension - 2 mm ) )"
equation "d440 = ( ( BaseY ) + ( ( ( Depth ) + DrainExtension - 2 mm ) + ( 1 mm ) ) )"
equation "d441 = -( -( ( FootHeight ) + ( 0.6 mm ) ) )"
equation "d442 = DrainWidth + 2 * Wall"
equation "d444 = FootHeight"
equation "d446 = ( BaseX + TowerWidth + ModuleGap ) + ( ( 11 mm ) - PegSize / 2 - FitClearance )"
equation "d447 = ( BaseY ) + ( ( 11 mm ) - PegSize / 2 - FitClearance )"
equation "d448 = PegSize + 2 * FitClearance"
equation "d449 = PegSize + 2 * FitClearance"
equation "d450 = PegHeight + 0.3 mm"
equation "d452 = FootHeight"
equation "d454 = ( BaseX + TowerWidth + ModuleGap ) + ( ( 11 mm ) - PegSize / 2 - FitClearance )"
equation "d455 = ( BaseY ) + ( ( ( Depth ) - FrontFootInset ) - PegSize / 2 - FitClearance )"
equation "d456 = PegSize + 2 * FitClearance"
equation "d457 = PegSize + 2 * FitClearance"
equation "d458 = PegHeight + 0.3 mm"
equation "d460 = FootHeight"
equation "d462 = ( BaseX + TowerWidth + ModuleGap ) + ( ( ( LeftRun - TowerWidth - ModuleGap ) - 11 mm ) - PegSize / 2 - FitClearance )"
equation "d463 = ( BaseY ) + ( ( 11 mm ) - PegSize / 2 - FitClearance )"
equation "d464 = PegSize + 2 * FitClearance"
equation "d465 = PegSize + 2 * FitClearance"
equation "d466 = PegHeight + 0.3 mm"
equation "d468 = FootHeight"
equation "d470 = ( BaseX + TowerWidth + ModuleGap ) + ( ( ( LeftRun - TowerWidth - ModuleGap ) - 11 mm ) - PegSize / 2 - FitClearance )"
equation "d471 = ( BaseY ) + ( ( ( Depth ) - FrontFootInset ) - PegSize / 2 - FitClearance )"
equation "d472 = PegSize + 2 * FitClearance"
equation "d473 = PegSize + 2 * FitClearance"
equation "d474 = PegHeight + 0.3 mm"
equation "d476 = ( FootHeight ) + PanHeight - DeckThick"
equation "d478 = ( BaseX + TowerWidth + ModuleGap ) + ( Wall + DeckClearance )"
equation "d479 = ( BaseY ) + ( Wall + DeckClearance )"
equation "d480 = ( LeftRun - TowerWidth - ModuleGap ) - 2 * ( Wall + DeckClearance )"
equation "d481 = ( Depth ) - 2 * ( Wall + DeckClearance )"
equation "d482 = DeckThick"
equation "d484 = ( FootHeight ) + PanHeight - DeckThick"
equation "d486 = ( BaseX + TowerWidth + ModuleGap ) + ( ( ( ( LeftRun - TowerWidth - ModuleGap ) - ( 16 * SlotPitch + SlotWidth ) ) / 2 ) + ( 0 * SlotPitch ) )"
equation "d487 = ( BaseY ) + ( Wall + DeckClearance + RimBorder )"
equation "d488 = SlotWidth"
equation "d489 = ( Depth ) - 2 * ( Wall + DeckClearance + RimBorder )"
equation "d490 = DeckThick"
equation "d492 = ( FootHeight ) + PanHeight - DeckThick"
equation "d494 = ( BaseX + TowerWidth + ModuleGap ) + ( ( ( ( LeftRun - TowerWidth - ModuleGap ) - ( 16 * SlotPitch + SlotWidth ) ) / 2 ) + ( 1 * SlotPitch ) )"
equation "d495 = ( BaseY ) + ( Wall + DeckClearance + RimBorder )"
equation "d496 = SlotWidth"
equation "d497 = ( Depth ) - 2 * ( Wall + DeckClearance + RimBorder )"
equation "d498 = DeckThick"
equation "d500 = ( FootHeight ) + PanHeight - DeckThick"
equation "d502 = ( BaseX + TowerWidth + ModuleGap ) + ( ( ( ( LeftRun - TowerWidth - ModuleGap ) - ( 16 * SlotPitch + SlotWidth ) ) / 2 ) + ( 2 * SlotPitch ) )"
equation "d503 = ( BaseY ) + ( Wall + DeckClearance + RimBorder )"
equation "d504 = SlotWidth"
equation "d505 = ( Depth ) - 2 * ( Wall + DeckClearance + RimBorder )"
equation "d506 = DeckThick"
equation "d508 = ( FootHeight ) + PanHeight - DeckThick"
equation "d510 = ( BaseX + TowerWidth + ModuleGap ) + ( ( ( ( LeftRun - TowerWidth - ModuleGap ) - ( 16 * SlotPitch + SlotWidth ) ) / 2 ) + ( 3 * SlotPitch ) )"
equation "d511 = ( BaseY ) + ( Wall + DeckClearance + RimBorder )"
equation "d512 = SlotWidth"
equation "d513 = ( Depth ) - 2 * ( Wall + DeckClearance + RimBorder )"
equation "d514 = DeckThick"
equation "d516 = ( FootHeight ) + PanHeight - DeckThick"
equation "d518 = ( BaseX + TowerWidth + ModuleGap ) + ( ( ( ( LeftRun - TowerWidth - ModuleGap ) - ( 16 * SlotPitch + SlotWidth ) ) / 2 ) + ( 4 * SlotPitch ) )"
equation "d519 = ( BaseY ) + ( Wall + DeckClearance + RimBorder )"
equation "d520 = SlotWidth"
equation "d521 = ( Depth ) - 2 * ( Wall + DeckClearance + RimBorder )"
equation "d522 = DeckThick"
equation "d524 = ( FootHeight ) + PanHeight - DeckThick"
equation "d526 = ( BaseX + TowerWidth + ModuleGap ) + ( ( ( ( LeftRun - TowerWidth - ModuleGap ) - ( 16 * SlotPitch + SlotWidth ) ) / 2 ) + ( 5 * SlotPitch ) )"
equation "d527 = ( BaseY ) + ( Wall + DeckClearance + RimBorder )"
equation "d528 = SlotWidth"
equation "d529 = ( Depth ) - 2 * ( Wall + DeckClearance + RimBorder )"
equation "d530 = DeckThick"
equation "d532 = ( FootHeight ) + PanHeight - DeckThick"
equation "d534 = ( BaseX + TowerWidth + ModuleGap ) + ( ( ( ( LeftRun - TowerWidth - ModuleGap ) - ( 16 * SlotPitch + SlotWidth ) ) / 2 ) + ( 6 * SlotPitch ) )"
equation "d535 = ( BaseY ) + ( Wall + DeckClearance + RimBorder )"
equation "d536 = SlotWidth"
equation "d537 = ( Depth ) - 2 * ( Wall + DeckClearance + RimBorder )"
equation "d538 = DeckThick"
equation "d540 = ( FootHeight ) + PanHeight - DeckThick"
equation "d542 = ( BaseX + TowerWidth + ModuleGap ) + ( ( ( ( LeftRun - TowerWidth - ModuleGap ) - ( 16 * SlotPitch + SlotWidth ) ) / 2 ) + ( 7 * SlotPitch ) )"
equation "d543 = ( BaseY ) + ( Wall + DeckClearance + RimBorder )"
equation "d544 = SlotWidth"
equation "d545 = ( Depth ) - 2 * ( Wall + DeckClearance + RimBorder )"
equation "d546 = DeckThick"
equation "d548 = ( FootHeight ) + PanHeight - DeckThick"
equation "d550 = ( BaseX + TowerWidth + ModuleGap ) + ( ( ( ( LeftRun - TowerWidth - ModuleGap ) - ( 16 * SlotPitch + SlotWidth ) ) / 2 ) + ( 8 * SlotPitch ) )"
equation "d551 = ( BaseY ) + ( Wall + DeckClearance + RimBorder )"
equation "d552 = SlotWidth"
equation "d553 = ( Depth ) - 2 * ( Wall + DeckClearance + RimBorder )"
equation "d554 = DeckThick"
equation "d556 = ( FootHeight ) + PanHeight - DeckThick"
equation "d558 = ( BaseX + TowerWidth + ModuleGap ) + ( ( ( ( LeftRun - TowerWidth - ModuleGap ) - ( 16 * SlotPitch + SlotWidth ) ) / 2 ) + ( 9 * SlotPitch ) )"
equation "d559 = ( BaseY ) + ( Wall + DeckClearance + RimBorder )"
equation "d560 = SlotWidth"
equation "d561 = ( Depth ) - 2 * ( Wall + DeckClearance + RimBorder )"
equation "d562 = DeckThick"
equation "d564 = ( FootHeight ) + PanHeight - DeckThick"
equation "d566 = ( BaseX + TowerWidth + ModuleGap ) + ( ( ( ( LeftRun - TowerWidth - ModuleGap ) - ( 16 * SlotPitch + SlotWidth ) ) / 2 ) + ( 10 * SlotPitch ) )"
equation "d567 = ( BaseY ) + ( Wall + DeckClearance + RimBorder )"
equation "d568 = SlotWidth"
equation "d569 = ( Depth ) - 2 * ( Wall + DeckClearance + RimBorder )"
equation "d570 = DeckThick"
equation "d572 = ( FootHeight ) + PanHeight - DeckThick"
equation "d574 = ( BaseX + TowerWidth + ModuleGap ) + ( ( ( ( LeftRun - TowerWidth - ModuleGap ) - ( 16 * SlotPitch + SlotWidth ) ) / 2 ) + ( 11 * SlotPitch ) )"
equation "d575 = ( BaseY ) + ( Wall + DeckClearance + RimBorder )"
equation "d576 = SlotWidth"
equation "d577 = ( Depth ) - 2 * ( Wall + DeckClearance + RimBorder )"
equation "d578 = DeckThick"
equation "d580 = ( FootHeight ) + PanHeight - DeckThick"
equation "d582 = ( BaseX + TowerWidth + ModuleGap ) + ( ( ( ( LeftRun - TowerWidth - ModuleGap ) - ( 16 * SlotPitch + SlotWidth ) ) / 2 ) + ( 12 * SlotPitch ) )"
equation "d583 = ( BaseY ) + ( Wall + DeckClearance + RimBorder )"
equation "d584 = SlotWidth"
equation "d585 = ( Depth ) - 2 * ( Wall + DeckClearance + RimBorder )"
equation "d586 = DeckThick"
equation "d588 = ( FootHeight ) + PanHeight - DeckThick"
equation "d590 = ( BaseX + TowerWidth + ModuleGap ) + ( ( ( ( LeftRun - TowerWidth - ModuleGap ) - ( 16 * SlotPitch + SlotWidth ) ) / 2 ) + ( 13 * SlotPitch ) )"
equation "d591 = ( BaseY ) + ( Wall + DeckClearance + RimBorder )"
equation "d592 = SlotWidth"
equation "d593 = ( Depth ) - 2 * ( Wall + DeckClearance + RimBorder )"
equation "d594 = DeckThick"
equation "d596 = ( FootHeight ) + PanHeight - DeckThick"
equation "d598 = ( BaseX + TowerWidth + ModuleGap ) + ( ( ( ( LeftRun - TowerWidth - ModuleGap ) - ( 16 * SlotPitch + SlotWidth ) ) / 2 ) + ( 14 * SlotPitch ) )"
equation "d599 = ( BaseY ) + ( Wall + DeckClearance + RimBorder )"
equation "d600 = SlotWidth"
equation "d601 = ( Depth ) - 2 * ( Wall + DeckClearance + RimBorder )"
equation "d602 = DeckThick"
equation "d604 = ( FootHeight ) + PanHeight - DeckThick"
equation "d606 = ( BaseX + TowerWidth + ModuleGap ) + ( ( ( ( LeftRun - TowerWidth - ModuleGap ) - ( 16 * SlotPitch + SlotWidth ) ) / 2 ) + ( 15 * SlotPitch ) )"
equation "d607 = ( BaseY ) + ( Wall + DeckClearance + RimBorder )"
equation "d608 = SlotWidth"
equation "d609 = ( Depth ) - 2 * ( Wall + DeckClearance + RimBorder )"
equation "d610 = DeckThick"
equation "d612 = ( FootHeight ) + PanHeight - DeckThick"
equation "d614 = ( BaseX + TowerWidth + ModuleGap ) + ( ( ( ( LeftRun - TowerWidth - ModuleGap ) - ( 16 * SlotPitch + SlotWidth ) ) / 2 ) + ( 16 * SlotPitch ) )"
equation "d615 = ( BaseY ) + ( Wall + DeckClearance + RimBorder )"
equation "d616 = SlotWidth"
equation "d617 = ( Depth ) - 2 * ( Wall + DeckClearance + RimBorder )"
equation "d618 = DeckThick"
equation "d620 = ( FootHeight ) + PanHeight - DeckThick"
equation "d622 = ( BaseX + TowerWidth + ModuleGap ) + ( ( LeftRun - TowerWidth - ModuleGap ) / 2 - 8 mm )"
equation "d623 = ( BaseY ) + ( ( Depth ) - Wall - DeckClearance - 4 mm )"
equation "d626 = DeckThick"
equation "d630 = ( BaseX + TowerWidth + ModuleGap ) + ( ( 11 mm ) - FootSize / 2 )"
equation "d631 = ( BaseY ) + ( ( 11 mm ) - FootSize / 2 )"
equation "d632 = FootSize"
equation "d633 = FootSize"
equation "d634 = FootHeight"
equation "d636 = FootHeight"
equation "d638 = ( BaseX + TowerWidth + ModuleGap ) + ( ( 11 mm ) - PegSize / 2 )"
equation "d639 = ( BaseY ) + ( ( 11 mm ) - PegSize / 2 )"
equation "d640 = PegSize"
equation "d641 = PegSize"
equation "d642 = PegHeight"
equation "d646 = ( BaseX + TowerWidth + ModuleGap ) + ( ( 11 mm ) - FootSize / 2 )"
equation "d647 = ( BaseY ) + ( ( ( Depth ) - FrontFootInset ) - FootSize / 2 )"
equation "d648 = FootSize"
equation "d649 = FootSize"
equation "d650 = FootHeight"
equation "d652 = FootHeight"
equation "d654 = ( BaseX + TowerWidth + ModuleGap ) + ( ( 11 mm ) - PegSize / 2 )"
equation "d655 = ( BaseY ) + ( ( ( Depth ) - FrontFootInset ) - PegSize / 2 )"
equation "d656 = PegSize"
equation "d657 = PegSize"
equation "d658 = PegHeight"
equation "d662 = ( BaseX + TowerWidth + ModuleGap ) + ( ( ( LeftRun - TowerWidth - ModuleGap ) - 11 mm ) - FootSize / 2 )"
equation "d663 = ( BaseY ) + ( ( 11 mm ) - FootSize / 2 )"
equation "d664 = FootSize"
equation "d665 = FootSize"
equation "d666 = FootHeight"
equation "d668 = FootHeight"
equation "d670 = ( BaseX + TowerWidth + ModuleGap ) + ( ( ( LeftRun - TowerWidth - ModuleGap ) - 11 mm ) - PegSize / 2 )"
equation "d671 = ( BaseY ) + ( ( 11 mm ) - PegSize / 2 )"
equation "d672 = PegSize"
equation "d673 = PegSize"
equation "d674 = PegHeight"
equation "d678 = ( BaseX + TowerWidth + ModuleGap ) + ( ( ( LeftRun - TowerWidth - ModuleGap ) - 11 mm ) - FootSize / 2 )"
equation "d679 = ( BaseY ) + ( ( ( Depth ) - FrontFootInset ) - FootSize / 2 )"
equation "d680 = FootSize"
equation "d681 = FootSize"
equation "d682 = FootHeight"
equation "d684 = FootHeight"
equation "d686 = ( BaseX + TowerWidth + ModuleGap ) + ( ( ( LeftRun - TowerWidth - ModuleGap ) - 11 mm ) - PegSize / 2 )"
equation "d687 = ( BaseY ) + ( ( ( Depth ) - FrontFootInset ) - PegSize / 2 )"
equation "d688 = PegSize"
equation "d689 = PegSize"
equation "d690 = PegHeight"
equation "d692 = FootHeight"
equation "d694 = ( BaseX + LeftRun + FaucetGap ) + ( 0 mm )"
equation "d695 = ( BaseY ) + ( 0 mm )"
equation "d696 = ( RightRun - ModuleGap ) / 2"
equation "d697 = Depth"
equation "d698 = PanHeight"